Autodesk Fusion 360 part; units mm, degrees
(part 3 of 4)
  line L2118 (-48.5, -68.866) -> (-48, -69.7321)
  line L2119 (-32, -63.7321) -> (-31.5, -62.866)
  line L2120 (-47, -75.7321) -> (-46.5, -74.866)
  line L2121 (-33, -75.7321) -> (-32, -75.7321)
  line L2122 (-46.5, -74.866) -> (-47, -74)
  line L2123 (-28.5, -65.866) -> (-29, -65)
  line L2124 (-45.5, -74.866) -> (-45, -75.7321)
  line L2125 (-33, -68) -> (-33.5, -68.866)
  line L2126 (-30, -66.7321) -> (-29, -66.7321)
  line L2127 (-45.5, -71.866) -> (-45, -72.7321)
  line L2128 (-29, -68) -> (-30, -68)
  line L2129 (-47, -72.7321) -> (-46.5, -71.866)
  line L2130 (-32, -65) -> (-33, -65)
  line L2131 (-45.5, -62.866) -> (-45, -63.7321)
  line L2132 (-29, -66.7321) -> (-28.5, -65.866)
  line L2133 (-48, -75.7321) -> (-47, -75.7321)
  line L2134 (-32, -66.7321) -> (-31.5, -65.866)
  line L2135 (-48.5, -59.866) -> (-48, -60.7321)
  line L2136 (-45, -68) -> (-45.5, -68.866)
  line L2137 (-48, -72.7321) -> (-47, -72.7321)
  line L2138 (-33, -63.7321) -> (-32, -63.7321)
  line L2139 (-33, -66.7321) -> (-32, -66.7321)
  line L2140 (-33, -65) -> (-33.5, -65.866)
  line L2141 (-30, -68) -> (-30.5, -68.866)
  line L2142 (-46.5, -68.866) -> (-47, -68)
  line L2143 (-47, -74) -> (-48, -74)
  line L2144 (-47, -68) -> (-48, -68)
  line L2145 (-33, -62) -> (-33.5, -62.866)
  line L2146 (-32, -68) -> (-33, -68)
  line L2147 (-48, -74) -> (-48.5, -74.866)
  line L2148 (-48.5, -71.866) -> (-48, -72.7321)
  line L2149 (-30.5, -62.866) -> (-30, -63.7321)
  line L2150 (-48, -71) -> (-48.5, -71.866)
  line L2151 (-28.5, -62.866) -> (-29, -62)
  line L2152 (-29, -65) -> (-30, -65)
  line L2153 (-47, -69.7321) -> (-46.5, -68.866)
  line L2154 (-29, -62) -> (-30, -62)
  line L2155 (-33.5, -65.866) -> (-33, -66.7321)
  line L2156 (-30, -65) -> (-30.5, -65.866)
  line L2157 (-31.5, -68.866) -> (-32, -68)
  line L2158 (-31.5, -65.866) -> (-32, -65)
  line L2159 (-48, -65) -> (-48.5, -65.866)
  line L2160 (-28.5, -68.866) -> (-29, -68)
  line L2161 (-47, -60.7321) -> (-46.5, -59.866)
  line L2162 (-45, -59) -> (-45.5, -59.866)
  line L2163 (-33, -60.7321) -> (-32, -60.7321)
  line L2164 (-30, -60.7321) -> (-29, -60.7321)
  line L2165 (-47, -59) -> (-48, -59)
  line L2166 (-46.5, -59.866) -> (-47, -59)
  line L2167 (-46.5, -62.866) -> (-47, -62)
  line L2168 (-48, -63.7321) -> (-47, -63.7321)
  line L2169 (-48, -66.7321) -> (-47, -66.7321)
  line L2170 (-45.5, -59.866) -> (-45, -60.7321)
  line L2171 (-32, -59) -> (-33, -59)
  line L2172 (-48.5, -65.866) -> (-48, -66.7321)
  line L2173 (-47, -66.7321) -> (-46.5, -65.866)
  line L2174 (-28.5, -59.866) -> (-29, -59)
  line L2175 (-46.5, -65.866) -> (-47, -65)
  line L2176 (-30.5, -59.866) -> (-30, -60.7321)
  line L2177 (-45, -65) -> (-45.5, -65.866)
  line L2178 (-33, -59) -> (-33.5, -59.866)
  line L2179 (-47, -62) -> (-48, -62)
  line L2180 (-29, -60.7321) -> (-28.5, -59.866)
  line L2181 (-48, -62) -> (-48.5, -62.866)
  line L2182 (-30, -59) -> (-30.5, -59.866)
  line L2183 (-45, -62) -> (-45.5, -62.866)
  line L2184 (-48, -60.7321) -> (-47, -60.7321)
  line L2185 (-31.5, -59.866) -> (-32, -59)
  line L2186 (-29, -59) -> (-30, -59)
  line L2187 (-32, -60.7321) -> (-31.5, -59.866)
  line L2188 (-33.5, -59.866) -> (-33, -60.7321)
  line L2189 (-48.5, -62.866) -> (-48, -63.7321)
  line L2190 (-45.5, -65.866) -> (-45, -66.7321)
  line L2191 (-48, -59) -> (-48.5, -59.866)
  line L2192 (-47, -63.7321) -> (-46.5, -62.866)
  line L2193 (-47, -65) -> (-48, -65)
  line L2194 (-42, -72.7321) -> (-41, -72.7321)
  line L2195 (-41, -74) -> (-42, -74)
  line L2196 (-24.5, -71.866) -> (-24, -72.7321)
  line L2197 (-41, -75.7321) -> (-40.5, -74.866)
  line L2198 (-41, -72.7321) -> (-40.5, -71.866)
  line L2199 (-40.5, -68.866) -> (-41, -68)
  line L2200 (-27, -69.7321) -> (-26, -69.7321)
  line L2201 (-41, -71) -> (-42, -71)
  line L2202 (-26, -69.7321) -> (-25.5, -68.866)
  line L2203 (-43.5, -74.866) -> (-44, -74)
  line L2204 (-39.5, -71.866) -> (-39, -72.7321)
  line L2205 (-54.5, -62.866) -> (-54, -63.7321)
  line L2206 (-54, -62) -> (-54.5, -62.866)
  line L2207 (-56, -59) -> (-57, -59)
  line L2208 (-35, -72.7321) -> (-34.5, -71.866)
  line L2209 (-38, -62) -> (-39, -62)
  line L2210 (-56, -62) -> (-57, -62)
  line L2211 (-38, -72.7321) -> (-37.5, -71.866)
  line L2212 (-56, -63.7321) -> (-55.5, -62.866)
  line L2213 (-57, -60.7321) -> (-56, -60.7321)
  line L2214 (-36, -75.7321) -> (-35, -75.7321)
  line L2215 (-34.5, -71.866) -> (-35, -71)
  line L2216 (-56, -66.7321) -> (-55.5, -65.866)
  line L2217 (-36, -66.7321) -> (-35, -66.7321)
  line L2218 (-57, -59) -> (-57.5, -59.866)
  line L2219 (-39.5, -68.866) -> (-39, -69.7321)
  line L2220 (-57, -62) -> (-57.5, -62.866)
  line L2221 (-57, -66.7321) -> (-56, -66.7321)
  line L2222 (-39, -66.7321) -> (-38, -66.7321)
  line L2223 (-36, -74) -> (-36.5, -74.866)
  line L2224 (-57.5, -65.866) -> (-57, -66.7321)
  line L2225 (-36, -63.7321) -> (-35, -63.7321)
  line L2226 (-35, -63.7321) -> (-34.5, -62.866)
  line L2227 (-36, -68) -> (-36.5, -68.866)
  line L2228 (-39.5, -65.866) -> (-39, -66.7321)
  line L2229 (-57.5, -62.866) -> (-57, -63.7321)
  line L2230 (-54.5, -59.866) -> (-54, -60.7321)
  line L2231 (-38, -63.7321) -> (-37.5, -62.866)
  line L2232 (-56, -60.7321) -> (-55.5, -59.866)
  line L2233 (-54, -59) -> (-54.5, -59.866)
  line L2234 (-54.5, -65.866) -> (-54, -66.7321)
  line L2235 (-36, -62) -> (-36.5, -62.866)
  line L2236 (-36.5, -71.866) -> (-36, -72.7321)
  line L2237 (-55.5, -65.866) -> (-56, -65)
  line L2238 (-34.5, -74.866) -> (-35, -74)
  line L2239 (-57, -63.7321) -> (-56, -63.7321)
  line L2240 (-35, -71) -> (-36, -71)
  line L2241 (-36.5, -74.866) -> (-36, -75.7321)
  line L2242 (-38, -69.7321) -> (-37.5, -68.866)
  line L2243 (-39, -69.7321) -> (-38, -69.7321)
  line L2244 (-35, -75.7321) -> (-34.5, -74.866)
  line L2245 (-55.5, -59.866) -> (-56, -59)
  line L2246 (-36.5, -68.866) -> (-36, -69.7321)
  line L2247 (-54, -65) -> (-54.5, -65.866)
  line L2248 (-38, -71) -> (-39, -71)
  line L2249 (-56, -65) -> (-57, -65)
  line L2250 (-39.5, -74.866) -> (-39, -75.7321)
  line L2251 (-39, -72.7321) -> (-38, -72.7321)
  line L2252 (-39, -74) -> (-39.5, -74.866)
  line L2253 (-39, -71) -> (-39.5, -71.866)
  line L2254 (-57.5, -59.866) -> (-57, -60.7321)
  line L2255 (-35, -74) -> (-36, -74)
  line L2256 (-35, -69.7321) -> (-34.5, -68.866)
  line L2257 (-57, -65) -> (-57.5, -65.866)
  line L2258 (-36, -72.7321) -> (-35, -72.7321)
  line L2259 (-55.5, -62.866) -> (-56, -62)
  line L2260 (-59, -72.7321) -> (-58.5, -71.866)
  line L2261 (-60, -75.7321) -> (-59, -75.7321)
  line L2262 (-59, -69.7321) -> (-58.5, -68.866)
  line L2263 (-59, -74) -> (-60, -74)
  line L2264 (-60, -74) -> (-60.5, -74.866)
  line L2265 (-63.5, -68.866) -> (-63, -69.7321)
  line L2266 (-61.5, -74.866) -> (-62, -74)
  line L2267 (-60.5, -71.866) -> (-60, -72.7321)
  line L2268 (-63.5, -74.866) -> (-63, -75.7321)
  line L2269 (-60.5, -68.866) -> (-60, -69.7321)
  line L2270 (-62, -75.7321) -> (-61.5, -74.866)
  line L2271 (-60, -69.7321) -> (-59, -69.7321)
  line L2272 (-63, -71) -> (-63.5, -71.866)
  line L2273 (-60, -72.7321) -> (-59, -72.7321)
  line L2274 (-60, -71) -> (-60.5, -71.866)
  line L2275 (-63, -72.7321) -> (-62, -72.7321)
  line L2276 (-60, -66.7321) -> (-59, -66.7321)
  line L2277 (-63, -65) -> (-63.5, -65.866)
  line L2278 (-63.5, -62.866) -> (-63, -63.7321)
  line L2279 (-59, -60.7321) -> (-58.5, -59.866)
  line L2280 (-59, -66.7321) -> (-58.5, -65.866)
  line L2281 (-60, -65) -> (-60.5, -65.866)
  line L2282 (-59, -65) -> (-60, -65)
  line L2283 (-60, -59) -> (-60.5, -59.866)
  line L2284 (-62, -66.7321) -> (-61.5, -65.866)
  line L2285 (-58.5, -62.866) -> (-59, -62)
  line L2286 (-63, -68) -> (-63.5, -68.866)
  line L2287 (-60.5, -65.866) -> (-60, -66.7321)
  line L2288 (-63.5, -59.866) -> (-63, -60.7321)
  line L2289 (-60, -63.7321) -> (-59, -63.7321)
  line L2290 (-62, -68) -> (-63, -68)
  line L2291 (-61.5, -65.866) -> (-62, -65)
  line L2292 (-60, -62) -> (-60.5, -62.866)
  line L2293 (-59, -63.7321) -> (-58.5, -62.866)
  line L2294 (-58.5, -68.866) -> (-59, -68)
  line L2295 (-63, -66.7321) -> (-62, -66.7321)
  line L2296 (-62, -62) -> (-63, -62)
  line L2297 (-59, -68) -> (-60, -68)
  line L2298 (-40.5, -74.866) -> (-41, -74)
  line L2299 (-25.5, -74.866) -> (-26, -74)
  line L2300 (-27, -74) -> (-27.5, -74.866)
  line L2301 (-42.5, -74.866) -> (-42, -75.7321)
  line L2302 (-44, -75.7321) -> (-43.5, -74.866)
  line L2303 (-42.5, -68.866) -> (-42, -69.7321)
  line L2304 (-26, -68) -> (-27, -68)
  line L2305 (-43.5, -68.866) -> (-44, -68)
  line L2306 (-42, -68) -> (-42.5, -68.866)
  line L2307 (-24.5, -68.866) -> (-24, -69.7321)
  line L2308 (-44, -69.7321) -> (-43.5, -68.866)
  line L2309 (-42, -75.7321) -> (-41, -75.7321)
  line L2310 (-40.5, -71.866) -> (-41, -71)
  line L2311 (-41, -68) -> (-42, -68)
  line L2312 (-25.5, -71.866) -> (-26, -71)
  line L2313 (-27.5, -71.866) -> (-27, -72.7321)
  line L2314 (-27.5, -68.866) -> (-27, -69.7321)
  line L2315 (-27, -72.7321) -> (-26, -72.7321)
  line L2316 (-26, -74) -> (-27, -74)
  line L2317 (-43.5, -71.866) -> (-44, -71)
  line L2318 (-42, -71) -> (-42.5, -71.866)
  line L2319 (-26, -75.7321) -> (-25.5, -74.866)
  line L2320 (-27, -75.7321) -> (-26, -75.7321)
  line L2321 (-26, -71) -> (-27, -71)
  line L2322 (-42.5, -71.866) -> (-42, -72.7321)
  line L2323 (-42, -74) -> (-42.5, -74.866)
  line L2324 (-24.5, -74.866) -> (-24, -75.7321)
  line L2325 (-42, -69.7321) -> (-41, -69.7321)
  line L2326 (-27, -71) -> (-27.5, -71.866)
  line L2327 (-24, -74) -> (-24.5, -74.866)
  line L2328 (-24, -71) -> (-24.5, -71.866)
  line L2329 (-27.5, -74.866) -> (-27, -75.7321)
  line L2330 (-41, -69.7321) -> (-40.5, -68.866)
  line L2331 (-26, -72.7321) -> (-25.5, -71.866)
  line L2332 (-44, -72.7321) -> (-43.5, -71.866)
  line L2333 (-26, -66.7321) -> (-25.5, -65.866)
  line L2334 (-27, -65) -> (-27.5, -65.866)
  line L2335 (-25.5, -68.866) -> (-26, -68)
  line L2336 (-41, -65) -> (-42, -65)
  line L2337 (-44, -66.7321) -> (-43.5, -65.866)
  line L2338 (-42, -65) -> (-42.5, -65.866)
  line L2339 (-27.5, -65.866) -> (-27, -66.7321)
  line L2340 (-26, -65) -> (-27, -65)
  line L2341 (-42.5, -62.866) -> (-42, -63.7321)
  line L2342 (-26, -62) -> (-27, -62)
  line L2343 (-42, -63.7321) -> (-41, -63.7321)
  line L2344 (-41, -62) -> (-42, -62)
  line L2345 (-25.5, -65.866) -> (-26, -65)
  line L2346 (-27.5, -62.866) -> (-27, -63.7321)
  line L2347 (-42, -59) -> (-42.5, -59.866)
  line L2348 (-24, -62) -> (-24.5, -62.866)
  line L2349 (-24.5, -62.866) -> (-24, -63.7321)
  line L2350 (-43.5, -59.866) -> (-44, -59)
  line L2351 (-27, -68) -> (-27.5, -68.866)
  line L2352 (-43.5, -65.866) -> (-44, -65)
  line L2353 (-27, -66.7321) -> (-26, -66.7321)
  line L2354 (-44, -60.7321) -> (-43.5, -59.866)
  line L2355 (-42.5, -65.866) -> (-42, -66.7321)
  line L2356 (-40.5, -62.866) -> (-41, -62)
  line L2357 (-24.5, -65.866) -> (-24, -66.7321)
  line L2358 (-24, -65) -> (-24.5, -65.866)
  line L2359 (-27, -63.7321) -> (-26, -63.7321)
  line L2360 (-42, -62) -> (-42.5, -62.866)
  line L2361 (-44, -63.7321) -> (-43.5, -62.866)
  line L2362 (-24, -68) -> (-24.5, -68.866)
  line L2363 (-42.5, -59.866) -> (-42, -60.7321)
  line L2364 (-41, -63.7321) -> (-40.5, -62.866)
  line L2365 (-41, -59) -> (-42, -59)
  line L2366 (-27, -62) -> (-27.5, -62.866)
  line L2367 (-42, -60.7321) -> (-41, -60.7321)
  line L2368 (-45, -66.7321) -> (-44, -66.7321)
  line L2369 (-26, -63.7321) -> (-25.5, -62.866)
  line L2370 (-44, -65) -> (-45, -65)
  line L2371 (-45, -75.7321) -> (-44, -75.7321)
  line L2372 (-25.5, -59.866) -> (-26, -59)
  line L2373 (-24.5, -59.866) -> (-24, -60.7321)
  line L2374 (-41, -66.7321) -> (-40.5, -65.866)
  line L2375 (-45, -69.7321) -> (-44, -69.7321)
  line L2376 (-24, -59) -> (-24.5, -59.866)
  line L2377 (-44, -68) -> (-45, -68)
  line L2378 (-26, -60.7321) -> (-25.5, -59.866)
  line L2379 (-27.5, -59.866) -> (-27, -60.7321)
  line L2380 (-42, -66.7321) -> (-41, -66.7321)
  line L2381 (-44, -74) -> (-45, -74)
  line L2382 (-20, -72.7321) -> (-19.5, -71.866)
  line L2383 (-45, -60.7321) -> (-44, -60.7321)
  line L2384 (-45, -72.7321) -> (-44, -72.7321)
  line L2385 (-26, -59) -> (-27, -59)
  line L2386 (-20, -74) -> (-21, -74)
  line L2387 (-25.5, -62.866) -> (-26, -62)
  line L2388 (-40.5, -65.866) -> (-41, -65)
  line L2389 (-40.5, -59.866) -> (-41, -59)
  line L2390 (-43.5, -62.866) -> (-44, -62)
  line L2391 (-41, -60.7321) -> (-40.5, -59.866)
  line L2392 (-44, -62) -> (-45, -62)
  line L2393 (-27, -60.7321) -> (-26, -60.7321)
  line L2394 (-45, -63.7321) -> (-44, -63.7321)
  line L2395 (-44, -59) -> (-45, -59)
  line L2396 (-27, -59) -> (-27.5, -59.866)
  line L2397 (-44, -71) -> (-45, -71)
  line L2398 (-21, -71) -> (-21.5, -71.866)
  line L2399 (-21, -72.7321) -> (-20, -72.7321)
  line L2400 (-20, -69.7321) -> (-19.5, -68.866)
  line L2401 (-21, -75.7321) -> (-20, -75.7321)
  line L2402 (-23, -75.7321) -> (-22.5, -74.866)
  line L2403 (-21.5, -71.866) -> (-21, -72.7321)
  line L2404 (-21.5, -68.866) -> (-21, -69.7321)
  line L2405 (-21.5, -74.866) -> (-21, -75.7321)
  line L2406 (-21, -69.7321) -> (-20, -69.7321)
  line L2407 (-24, -66.7321) -> (-23, -66.7321)
  line L2408 (-16.5, -65.866) -> (-17, -65)
  line L2409 (-17, -60.7321) -> (-16.5, -59.866)
  line L2410 (-18, -62) -> (-18.5, -62.866)
  line L2411 (-24, -75.7321) -> (-23, -75.7321)
  line L2412 (-15, -62) -> (-15.5, -62.866)
  line L2413 (-18, -65) -> (-18.5, -65.866)
  line L2414 (-15, -65) -> (-15.5, -65.866)
  line L2415 (-23, -65) -> (-24, -65)
  line L2416 (-17, -63.7321) -> (-16.5, -62.866)
  line L2417 (-18, -60.7321) -> (-17, -60.7321)
  line L2418 (-18, -68) -> (-18.5, -68.866)
  line L2419 (-15.5, -59.866) -> (-15, -60.7321)
  line L2420 (-24, -69.7321) -> (-23, -69.7321)
  line L2421 (-18, -63.7321) -> (-17, -63.7321)
  line L2422 (-16.5, -68.866) -> (-17, -68)
  line L2423 (-15.5, -65.866) -> (-15, -66.7321)
  line L2424 (-17, -68) -> (-18, -68)
  line L2425 (-18, -59) -> (-18.5, -59.866)
  line L2426 (-22.5, -74.866) -> (-23, -74)
  line L2427 (-21.5, -62.866) -> (-21, -63.7321)
  line L2428 (-20, -71) -> (-21, -71)
  line L2429 (-22.5, -71.866) -> (-23, -71)
  line L2430 (-19.5, -74.866) -> (-20, -74)
  line L2431 (-21, -68) -> (-21.5, -68.866)
  line L2432 (-19.5, -71.866) -> (-20, -71)
  line L2433 (-22.5, -62.866) -> (-23, -62)
  line L2434 (-15, -74) -> (-15.5, -74.866)
  line L2435 (-19.5, -68.866) -> (-20, -68)
  line L2436 (-20, -68) -> (-21, -68)
  line L2437 (-23, -72.7321) -> (-22.5, -71.866)
  line L2438 (-20, -75.7321) -> (-19.5, -74.866)
  line L2439 (-21, -62) -> (-21.5, -62.866)
  line L2440 (-23, -69.7321) -> (-22.5, -68.866)
  line L2441 (-21, -74) -> (-21.5, -74.866)
  line L2442 (-17, -75.7321) -> (-16.5, -74.866)
  line L2443 (-20, -66.7321) -> (-19.5, -65.866)
  line L2444 (-18, -69.7321) -> (-17, -69.7321)
  line L2445 (-19.5, -62.866) -> (-20, -62)
  line L2446 (-18.5, -71.866) -> (-18, -72.7321)
  line L2447 (-18, -74) -> (-18.5, -74.866)
  line L2448 (-15, -71) -> (-15.5, -71.866)
  line L2449 (-21, -59) -> (-21.5, -59.866)
  line L2450 (-17, -72.7321) -> (-16.5, -71.866)
  line L2451 (-20, -59) -> (-21, -59)
  line L2452 (-22.5, -65.866) -> (-23, -65)
  line L2453 (-21.5, -65.866) -> (-21, -66.7321)
  line L2454 (-21, -63.7321) -> (-20, -63.7321)
  line L2455 (-17, -74) -> (-18, -74)
  line L2456 (-21, -66.7321) -> (-20, -66.7321)
  line L2457 (-23, -63.7321) -> (-22.5, -62.866)
  line L2458 (-20, -62) -> (-21, -62)
  line L2459 (-15.5, -74.866) -> (-15, -75.7321)
  line L2460 (-18, -71) -> (-18.5, -71.866)
  line L2461 (-16.5, -71.866) -> (-17, -71)
  line L2462 (-19.5, -65.866) -> (-20, -65)
  line L2463 (-19.5, -59.866) -> (-20, -59)
  line L2464 (-18.5, -68.866) -> (-18, -69.7321)
  line L2465 (-23, -60.7321) -> (-22.5, -59.866)
  line L2466 (-18.5, -62.866) -> (-18, -63.7321)
  line L2467 (-20, -65) -> (-21, -65)
  line L2468 (-16.5, -74.866) -> (-17, -74)
  line L2469 (-18, -75.7321) -> (-17, -75.7321)
  line L2470 (-17, -71) -> (-18, -71)
  line L2471 (-15.5, -68.866) -> (-15, -69.7321)
  line L2472 (-21, -65) -> (-21.5, -65.866)
  line L2473 (-20, -63.7321) -> (-19.5, -62.866)
  line L2474 (-15.5, -71.866) -> (-15, -72.7321)
  line L2475 (-18, -72.7321) -> (-17, -72.7321)
  line L2476 (-22.5, -68.866) -> (-23, -68)
  line L2477 (-18.5, -74.866) -> (-18, -75.7321)
  line L2478 (-17, -69.7321) -> (-16.5, -68.866)
  line L2479 (-23, -66.7321) -> (-22.5, -65.866)
  line L2480 (-22.5, -59.866) -> (-23, -59)
  line L2481 (-20, -60.7321) -> (-19.5, -59.866)
  line L2482 (-17, -65) -> (-18, -65)
  line L2483 (-17, -62) -> (-18, -62)
  line L2484 (-15.5, -62.866) -> (-15, -63.7321)
  line L2485 (-24, -63.7321) -> (-23, -63.7321)
  line L2486 (-16.5, -62.866) -> (-17, -62)
  line L2487 (-23, -59) -> (-24, -59)
  line L2488 (-15, -68) -> (-15.5, -68.866)
  line L2489 (-23, -62) -> (-24, -62)
  line L2490 (-23, -71) -> (-24, -71)
  line L2491 (-21, -60.7321) -> (-20, -60.7321)
  line L2492 (-24, -60.7321) -> (-23, -60.7321)
  line L2493 (-24, -72.7321) -> (-23, -72.7321)
  line L2494 (-23, -68) -> (-24, -68)
  line L2495 (-18.5, -65.866) -> (-18, -66.7321)
  line L2496 (-21.5, -59.866) -> (-21, -60.7321)
  line L2497 (-23, -74) -> (-24, -74)
  line L2498 (-18, -66.7321) -> (-17, -66.7321)
  line L2499 (-17, -66.7321) -> (-16.5, -65.866)
  line L2500 (-49.5, -65.866) -> (-50, -65)
  line L2501 (-37.5, -68.866) -> (-38, -68)
  line L2502 (-39, -60.7321) -> (-38, -60.7321)
  line L2503 (-51.5, -65.866) -> (-51, -66.7321)
  line L2504 (-34.5, -59.866) -> (-35, -59)
  line L2505 (-38, -59) -> (-39, -59)
  line L2506 (-50, -59) -> (-51, -59)
  line L2507 (-36.5, -65.866) -> (-36, -66.7321)
  line L2508 (-51, -74) -> (-51.5, -74.866)
  line L2509 (-52.5, -68.866) -> (-53, -68)
  line L2510 (-49.5, -68.866) -> (-50, -68)
  line L2511 (-53, -72.7321) -> (-52.5, -71.866)
  line L2512 (-35, -66.7321) -> (-34.5, -65.866)
  line L2513 (-35, -65) -> (-36, -65)
  line L2514 (-50, -75.7321) -> (-49.5, -74.866)
  line L2515 (-51, -69.7321) -> (-50, -69.7321)
  line L2516 (-52.5, -71.866) -> (-53, -71)
  line L2517 (-35, -60.7321) -> (-34.5, -59.866)
  line L2518 (-39, -65) -> (-39.5, -65.866)
  line L2519 (-36, -59) -> (-36.5, -59.866)
  line L2520 (-35, -59) -> (-36, -59)
  line L2521 (-37.5, -62.866) -> (-38, -62)
  line L2522 (-39, -68) -> (-39.5, -68.866)
  line L2523 (-51.5, -68.866) -> (-51, -69.7321)
  line L2524 (-53, -60.7321) -> (-52.5, -59.866)
  line L2525 (-51.5, -74.866) -> (-51, -75.7321)
  line L2526 (-39, -59) -> (-39.5, -59.866)
  line L2527 (-36.5, -59.866) -> (-36, -60.7321)
  line L2528 (-50, -62) -> (-51, -62)
  line L2529 (-38, -60.7321) -> (-37.5, -59.866)
  line L2530 (-49.5, -74.866) -> (-50, -74)
  line L2531 (-49.5, -71.866) -> (-50, -71)
  line L2532 (-35, -62) -> (-36, -62)
  line L2533 (-38, -68) -> (-39, -68)
  line L2534 (-36, -65) -> (-36.5, -65.866)
  line L2535 (-36.5, -62.866) -> (-36, -63.7321)
  line L2536 (-53, -69.7321) -> (-52.5, -68.866)
  line L2537 (-34.5, -68.866) -> (-35, -68)
  line L2538 (-50, -72.7321) -> (-49.5, -71.866)
  line L2539 (-51, -68) -> (-51.5, -68.866)
  line L2540 (-35, -68) -> (-36, -68)
  line L2541 (-51, -71) -> (-51.5, -71.866)
  line L2542 (-37.5, -65.866) -> (-38, -65)
  line L2543 (-50, -68) -> (-51, -68)
  line L2544 (-39, -63.7321) -> (-38, -63.7321)
  line L2545 (-50, -74) -> (-51, -74)
  line L2546 (-38, -66.7321) -> (-37.5, -65.866)
  line L2547 (-34.5, -65.866) -> (-35, -65)
  line L2548 (-39.5, -62.866) -> (-39, -63.7321)
  line L2549 (-51, -75.7321) -> (-50, -75.7321)
  line L2550 (-50, -69.7321) -> (-49.5, -68.866)
  line L2551 (-51.5, -71.866) -> (-51, -72.7321)
  line L2552 (-52.5, -74.866) -> (-53, -74)
  line L2553 (-39, -62) -> (-39.5, -62.866)
  line L2554 (-38, -65) -> (-39, -65)
  line L2555 (-50, -71) -> (-51, -71)
  line L2556 (-34.5, -62.866) -> (-35, -62)
  line L2557 (-51, -72.7321) -> (-50, -72.7321)
  line L2558 (-53, -75.7321) -> (-52.5, -74.866)
  line L2559 (-51, -60.7321) -> (-50, -60.7321)
  line L2560 (-32, -71) -> (-33, -71)
  line L2561 (-32, -72.7321) -> (-31.5, -71.866)
  line L2562 (-30.5, -71.866) -> (-30, -72.7321)
  line L2563 (-51.5, -59.866) -> (-51, -60.7321)
  line L2564 (-49.5, -62.866) -> (-50, -62)
  line L2565 (-36, -60.7321) -> (-35, -60.7321)
  line L2566 (-52.5, -65.866) -> (-53, -65)
  line L2567 (-37.5, -59.866) -> (-38, -59)
  line L2568 (-51.5, -62.866) -> (-51, -63.7321)
  line L2569 (-52.5, -59.866) -> (-53, -59)
  line L2570 (-51, -59) -> (-51.5, -59.866)
  line L2571 (-33, -71) -> (-33.5, -71.866)
  line L2572 (-30.5, -74.866) -> (-30, -75.7321)
  line L2573 (-51, -66.7321) -> (-50, -66.7321)
  line L2574 (-52.5, -62.866) -> (-53, -62)
  line L2575 (-51, -62) -> (-51.5, -62.866)
  line L2576 (-29, -75.7321) -> (-28.5, -74.866)
  line L2577 (-53, -71) -> (-54, -71)
  line L2578 (-53, -66.7321) -> (-52.5, -65.866)
  line L2579 (-30, -69.7321) -> (-29, -69.7321)
  line L2580 (-51, -63.7321) -> (-50, -63.7321)
  line L2581 (-51, -65) -> (-51.5, -65.866)
  line L2582 (-50, -65) -> (-51, -65)
  line L2583 (-50, -66.7321) -> (-49.5, -65.866)
  line L2584 (-39.5, -59.866) -> (-39, -60.7321)
  line L2585 (-49.5, -59.866) -> (-50, -59)
  line L2586 (-29, -71) -> (-30, -71)
  line L2587 (-50, -63.7321) -> (-49.5, -62.866)
  line L2588 (-32, -74) -> (-33, -74)
  line L2589 (-50, -60.7321) -> (-49.5, -59.866)
  line L2590 (-53, -63.7321) -> (-52.5, -62.866)
  line L2591 (-30, -72.7321) -> (-29, -72.7321)
  line L2592 (-33.5, -71.866) -> (-33, -72.7321)
  line L2593 (-53, -59) -> (-54, -59)
  line L2594 (-54, -63.7321) -> (-53, -63.7321)
  line L2595 (-53, -65) -> (-54, -65)
  line L2596 (-31.5, -74.866) -> (-32, -74)
  line L2597 (-53, -74) -> (-54, -74)
  line L2598 (-54, -72.7321) -> (-53, -72.7321)
  line L2599 (-53, -62) -> (-54, -62)
  line L2600 (-28.5, -74.866) -> (-29, -74)
  line L2601 (-30.5, -68.866) -> (-30, -69.7321)
  line L2602 (-28.5, -71.866) -> (-29, -71)
  line L2603 (-33, -72.7321) -> (-32, -72.7321)
  line L2604 (-29, -69.7321) -> (-28.5, -68.866)
  line L2605 (-32, -75.7321) -> (-31.5, -74.866)
  line L2606 (-54, -66.7321) -> (-53, -66.7321)
  line L2607 (-30, -74) -> (-30.5, -74.866)
  line L2608 (-32, -69.7321) -> (-31.5, -68.866)
  line L2609 (-30, -71) -> (-30.5, -71.866)
  line L2610 (-54, -69.7321) -> (-53, -69.7321)
  line L2611 (-54, -60.7321) -> (-53, -60.7321)
  line L2612 (-30, -75.7321) -> (-29, -75.7321)
  line L2613 (-33, -74) -> (-33.5, -74.866)
  line L2614 (-54, -75.7321) -> (-53, -75.7321)
  line L2615 (-33.5, -74.866) -> (-33, -75.7321)
  line L2616 (-31.5, -71.866) -> (-32, -71)
  line L2617 (-53, -68) -> (-54, -68)
  line L2618 (-29, -74) -> (-30, -74)
  line L2619 (-17, -59) -> (-18, -59)
  line L2620 (-15, -59) -> (-15.5, -59.866)
  line L2621 (-18.5, -59.866) -> (-18, -60.7321)
  line L2622 (-16.5, -59.866) -> (-17, -59)
  line L2623 (-63.5, -65.866) -> (-63, -66.7321)
  line L2624 (-63, -63.7321) -> (-62, -63.7321)
  line L2625 (-59, -62) -> (-60, -62)
  line L2626 (-63, -62) -> (-63.5, -62.866)
  line L2627 (-61.5, -68.866) -> (-62, -68)
  line L2628 (-62, -65) -> (-63, -65)
  line L2629 (-62, -63.7321) -> (-61.5, -62.866)
  line L2630 (-60, -68) -> (-60.5, -68.866)
  line L2631 (-61.5, -62.866) -> (-62, -62)
  line L2632 (-58.5, -65.866) -> (-59, -65)
  line L2633 (-60.5, -62.866) -> (-60, -63.7321)
  line L2634 (-61.5, -71.866) -> (-62, -71)
  line L2635 (-58.5, -74.866) -> (-59, -74)
  line L2636 (-63, -69.7321) -> (-62, -69.7321)
  line L2637 (-58.5, -71.866) -> (-59, -71)
  line L2638 (-63, -75.7321) -> (-62, -75.7321)
  line L2639 (-63, -74) -> (-63.5, -74.866)
  line L2640 (-63.5, -71.866) -> (-63, -72.7321)
  line L2641 (-59, -71) -> (-60, -71)
  line L2642 (-62, -71) -> (-63, -71)
  line L2643 (-62, -69.7321) -> (-61.5, -68.866)
  line L2644 (-12.5, -80.866) -> (-12, -81.7321)
  line L2645 (-10.5, -80.866) -> (-11, -80)
  line L2646 (-12, -77) -> (-12.5, -77.866)
  line L2647 (-17, -78.7321) -> (-16.5, -77.866)
  line L2648 (-44, -80) -> (-45, -80)
  line L2649 (-18, -78.7321) -> (-17, -78.7321)
  line L2650 (-22.5, -80.866) -> (-23, -80)
  line L2651 (-41, -77) -> (-42, -77)
  line L2652 (-21, -80) -> (-21.5, -80.866)
  line L2653 (-20, -81.7321) -> (-19.5, -80.866)
  line L2654 (-44, -78.7321) -> (-43.5, -77.866)
  line L2655 (-16.5, -80.866) -> (-17, -80)
  line L2656 (-21, -77) -> (-21.5, -77.866)
  line L2657 (-41, -81.7321) -> (-40.5, -80.866)
  line L2658 (-12.5, -77.866) -> (-12, -78.7321)
  line L2659 (-23, -77) -> (-24, -77)
  line L2660 (-20, -77) -> (-21, -77)
  line L2661 (-22.5, -77.866) -> (-23, -77)
  line L2662 (-24, -78.7321) -> (-23, -78.7321)
  line L2663 (-23, -78.7321) -> (-22.5, -77.866)
  line L2664 (-23, -80) -> (-24, -80)
  line L2665 (-44, -81.7321) -> (-43.5, -80.866)
  line L2666 (-20, -78.7321) -> (-19.5, -77.866)
  line L2667 (-20, -80) -> (-21, -80)
  line L2668 (-42, -77) -> (-42.5, -77.866)
  line L2669 (-42, -81.7321) -> (-41, -81.7321)
  line L2670 (-15.5, -77.866) -> (-15, -78.7321)
  line L2671 (-18, -80) -> (-18.5, -80.866)
  line L2672 (-42, -80) -> (-42.5, -80.866)
  line L2673 (-21, -78.7321) -> (-20, -78.7321)
  line L2674 (-17, -80) -> (-18, -80)
  line L2675 (-21.5, -77.866) -> (-21, -78.7321)
  line L2676 (-40.5, -77.866) -> (-41, -77)
  line L2677 (-15.5, -80.866) -> (-15, -81.7321)
  line L2678 (-19.5, -80.866) -> (-20, -80)
  line L2679 (-18.5, -80.866) -> (-18, -81.7321)
  line L2680 (-15, -77) -> (-15.5, -77.866)
  line L2681 (-40.5, -80.866) -> (-41, -80)
  line L2682 (-17, -77) -> (-18, -77)
  line L2683 (-12, -80) -> (-12.5, -80.866)
  line L2684 (-11, -81.7321) -> (-10.5, -80.866)
  line L2685 (-11, -80) -> (-12, -80)
  line L2686 (-21.5, -80.866) -> (-21, -81.7321)
  line L2687 (-18, -81.7321) -> (-17, -81.7321)
  line L2688 (-24, -81.7321) -> (-23, -81.7321)
  line L2689 (-45, -78.7321) -> (-44, -78.7321)
  line L2690 (-21, -81.7321) -> (-20, -81.7321)
  line L2691 (-23, -81.7321) -> (-22.5, -80.866)
  line L2692 (-18, -77) -> (-18.5, -77.866)
  line L2693 (-44, -77) -> (-45, -77)
  line L2694 (-19.5, -77.866) -> (-20, -77)
  line L2695 (-10.5, -77.866) -> (-11, -77)
  line L2696 (-14, -78.7321) -> (-13.5, -77.866)
  line L2697 (-13.5, -77.866) -> (-14, -77)
  line L2698 (-11, -77) -> (-12, -77)
  line L2699 (-11, -78.7321) -> (-10.5, -77.866)
  line L2700 (-12, -78.7321) -> (-11, -78.7321)
  line L2701 (-13.5, -80.866) -> (-14, -80)
  line L2702 (-12, -81.7321) -> (-11, -81.7321)
  line L2703 (-14, -77) -> (-15, -77)
  line L2704 (-15, -81.7321) -> (-14, -81.7321)
  line L2705 (-14, -81.7321) -> (-13.5, -80.866)
  line L2706 (-15, -78.7321) -> (-14, -78.7321)
  line L2707 (-14, -80) -> (-15, -80)
  line L2708 (-35, -81.7321) -> (-34.5, -80.866)
  line L2709 (-57, -80) -> (-57.5, -80.866)
  line L2710 (-35, -77) -> (-36, -77)
  line L2711 (-57, -77) -> (-57.5, -77.866)
  line L2712 (-54, -77) -> (-54.5, -77.866)
  line L2713 (-63, -78.7321) -> (-62, -78.7321)
  line L2714 (-60.5, -77.866) -> (-60, -78.7321)
  line L2715 (-59, -81.7321) -> (-58.5, -80.866)
  line L2716 (-63, -80) -> (-63.5, -80.866)
  line L2717 (-63.5, -77.866) -> (-63, -78.7321)
  line L2718 (-63, -81.7321) -> (-62, -81.7321)
  line L2719 (-60, -77) -> (-60.5, -77.866)
  line L2720 (-59, -80) -> (-60, -80)
  line L2721 (-60.5, -80.866) -> (-60, -81.7321)
  line L2722 (-59, -77) -> (-60, -77)
  line L2723 (-62, -78.7321) -> (-61.5, -77.866)
  line L2724 (-62, -80) -> (-63, -80)
  line L2725 (-61.5, -77.866) -> (-62, -77)
  line L2726 (-58.5, -77.866) -> (-59, -77)
  line L2727 (-63.5, -80.866) -> (-63, -81.7321)
  line L2728 (-60, -78.7321) -> (-59, -78.7321)
  line L2729 (-62, -77) -> (-63, -77)
  line L2730 (-60, -81.7321) -> (-59, -81.7321)
  line L2731 (-63, -77) -> (-63.5, -77.866)
  line L2732 (-61.5, -80.866) -> (-62, -80)
  line L2733 (-62, -81.7321) -> (-61.5, -80.866)
  line L2734 (-58.5, -80.866) -> (-59, -80)
  line L2735 (-60, -80) -> (-60.5, -80.866)
  line L2736 (-59, -78.7321) -> (-58.5, -77.866)
  line L2737 (-68, -77) -> (-69, -77)
  line L2738 (-69, -77) -> (-69.5, -77.866)
  line L2739 (-65, -78.7321) -> (-64.5, -77.866)
  line L2740 (-66, -81.7321) -> (-65, -81.7321)
  line L2741 (-69, -81.7321) -> (-68, -81.7321)
  line L2742 (-66.5, -77.866) -> (-66, -78.7321)
  line L2743 (-68, -81.7321) -> (-67.5, -80.866)
  line L2744 (-66, -80) -> (-66.5, -80.866)
  line L2745 (-66, -77) -> (-66.5, -77.866)
  line L2746 (-65, -77) -> (-66, -77)
  line L2747 (-68, -80) -> (-69, -80)
  line L2748 (-65, -81.7321) -> (-64.5, -80.866)
  line L2749 (-66.5, -80.866) -> (-66, -81.7321)
  line L2750 (-65, -80) -> (-66, -80)
  line L2751 (-66, -78.7321) -> (-65, -78.7321)
  line L2752 (-64.5, -77.866) -> (-65, -77)
  line L2753 (-69.5, -80.866) -> (-69, -81.7321)
  line L2754 (-69.5, -77.866) -> (-69, -78.7321)
  line L2755 (-67.5, -80.866) -> (-68, -80)
  line L2756 (-69, -78.7321) -> (-68, -78.7321)
  line L2757 (-68, -78.7321) -> (-67.5, -77.866)
  line L2758 (-69, -80) -> (-69.5, -80.866)
  line L2759 (-64.5, -80.866) -> (-65, -80)
  line L2760 (-57.5, -77.866) -> (-57, -78.7321)
  line L2761 (-57, -78.7321) -> (-56, -78.7321)
  line L2762 (-56, -78.7321) -> (-55.5, -77.866)
  line L2763 (-39.5, -80.866) -> (-39, -81.7321)
  line L2764 (-55.5, -80.866) -> (-56, -80)
  line L2765 (-39, -81.7321) -> (-38, -81.7321)
  line L2766 (-38, -77) -> (-39, -77)
  line L2767 (-55.5, -77.866) -> (-56, -77)
  line L2768 (-56, -81.7321) -> (-55.5, -80.866)
  line L2769 (-56, -77) -> (-57, -77)
  line L2770 (-54.5, -80.866) -> (-54, -81.7321)
  line L2771 (-67.5, -77.866) -> (-68, -77)
  line L2772 (-36, -78.7321) -> (-35, -78.7321)
  line L2773 (-57, -81.7321) -> (-56, -81.7321)
  line L2774 (-54, -80) -> (-54.5, -80.866)
  line L2775 (-35, -80) -> (-36, -80)
  line L2776 (-57.5, -80.866) -> (-57, -81.7321)
  line L2777 (-54.5, -77.866) -> (-54, -78.7321)
  line L2778 (-39, -78.7321) -> (-38, -78.7321)
  line L2779 (-56, -80) -> (-57, -80)
  line L2780 (-51.5, -77.866) -> (-51, -78.7321)
  line L2781 (-54, -78.7321) -> (-53, -78.7321)
  line L2782 (-39.5, -77.866) -> (-39, -78.7321)
  line L2783 (-50, -81.7321) -> (-49.5, -80.866)
  line L2784 (-33, -78.7321) -> (-32, -78.7321)
  line L2785 (-53, -81.7321) -> (-52.5, -80.866)
  line L2786 (-53, -80) -> (-54, -80)
  line L2787 (-33.5, -77.866) -> (-33, -78.7321)
  line L2788 (-30.5, -77.866) -> (-30, -78.7321)
  line L2789 (-31.5, -77.866) -> (-32, -77)
  line L2790 (-30, -81.7321) -> (-29, -81.7321)
  line L2791 (-30, -80) -> (-30.5, -80.866)
  line L2792 (-28.5, -80.866) -> (-29, -80)
  line L2793 (-49.5, -80.866) -> (-50, -80)
  line L2794 (-51, -80) -> (-51.5, -80.866)
  line L2795 (-36, -80) -> (-36.5, -80.866)
  line L2796 (-50, -78.7321) -> (-49.5, -77.866)
  line L2797 (-36, -81.7321) -> (-35, -81.7321)
  line L2798 (-49.5, -77.866) -> (-50, -77)
  line L2799 (-36, -77) -> (-36.5, -77.866)
  line L2800 (-51, -81.7321) -> (-50, -81.7321)
  line L2801 (-36.5, -77.866) -> (-36, -78.7321)
  line L2802 (-51.5, -80.866) -> (-51, -81.7321)
  line L2803 (-35, -78.7321) -> (-34.5, -77.866)
  line L2804 (-51, -77) -> (-51.5, -77.866)
  line L2805 (-50, -80) -> (-51, -80)
  line L2806 (-50, -77) -> (-51, -77)
  line L2807 (-37.5, -80.866) -> (-38, -80)
  line L2808 (-51, -78.7321) -> (-50, -78.7321)
  line L2809 (-53, -78.7321) -> (-52.5, -77.866)
  line L2810 (-39, -80) -> (-39.5, -80.866)
  line L2811 (-52.5, -77.866) -> (-53, -77)
  line L2812 (-52.5, -80.866) -> (-53, -80)
  line L2813 (-53, -77) -> (-54, -77)
  line L2814 (-54, -81.7321) -> (-53, -81.7321)
  line L2815 (-33, -80) -> (-33.5, -80.866)
  line L2816 (-30, -77) -> (-30.5, -77.866)
  line L2817 (-29, -81.7321) -> (-28.5, -80.866)
  line L2818 (-33, -81.7321) -> (-32, -81.7321)
  line L2819 (-32, -80) -> (-33, -80)
  line L2820 (-47, -77) -> (-48, -77)
  line L2821 (-30, -78.7321) -> (-29, -78.7321)
  line L2822 (-30.5, -80.866) -> (-30, -81.7321)
  line L2823 (-32, -81.7321) -> (-31.5, -80.866)
  line L2824 (-46.5, -80.866) -> (-47, -80)
  line L2825 (-29, -78.7321) -> (-28.5, -77.866)
  line L2826 (-31.5, -80.866) -> (-32, -80)
  line L2827 (-45, -81.7321) -> (-44, -81.7321)
  line L2828 (-45.5, -77.866) -> (-45, -78.7321)
  line L2829 (-32, -77) -> (-33, -77)
  line L2830 (-33.5, -80.866) -> (-33, -81.7321)
  line L2831 (-45, -80) -> (-45.5, -80.866)
  line L2832 (-29, -80) -> (-30, -80)
  line L2833 (-48.5, -77.866) -> (-48, -78.7321)
  line L2834 (-28.5, -77.866) -> (-29, -77)
  line L2835 (-46.5, -77.866) -> (-47, -77)
  line L2836 (-33, -77) -> (-33.5, -77.866)
  line L2837 (-42.5, -77.866) -> (-42, -78.7321)
  line L2838 (-18.5, -77.866) -> (-18, -78.7321)
  line L2839 (-47, -81.7321) -> (-46.5, -80.866)
  line L2840 (-43.5, -80.866) -> (-44, -80)
  line L2841 (-45, -77) -> (-45.5, -77.866)
  line L2842 (-26, -81.7321) -> (-25.5, -80.866)
  line L2843 (-47, -78.7321) -> (-46.5, -77.866)
  line L2844 (-48, -78.7321) -> (-47, -78.7321)
  line L2845 (-26, -78.7321) -> (-25.5, -77.866)
  line L2846 (-48, -81.7321) -> (-47, -81.7321)
  line L2847 (-25.5, -77.866) -> (-26, -77)
  line L2848 (-25.5, -80.866) -> (-26, -80)
  line L2849 (-42.5, -80.866) -> (-42, -81.7321)
  line L2850 (-15, -80) -> (-15.5, -80.866)
  line L2851 (-43.5, -77.866) -> (-44, -77)
  line L2852 (-41, -78.7321) -> (-40.5, -77.866)
  line L2853 (-47, -80) -> (-48, -80)
  line L2854 (-24, -80) -> (-24.5, -80.866)
  line L2855 (-24.5, -77.866) -> (-24, -78.7321)
  line L2856 (-29, -77) -> (-30, -77)
  line L2857 (-24.5, -80.866) -> (-24, -81.7321)
  line L2858 (-27, -81.7321) -> (-26, -81.7321)
  line L2859 (-26, -77) -> (-27, -77)
  line L2860 (-45.5, -80.866) -> (-45, -81.7321)
  line L2861 (-32, -78.7321) -> (-31.5, -77.866)
  line L2862 (-48, -77) -> (-48.5, -77.866)
  line L2863 (-27, -77) -> (-27.5, -77.866)
  line L2864 (-27, -78.7321) -> (-26, -78.7321)
  line L2865 (-27, -80) -> (-27.5, -80.866)
  line L2866 (-26, -80) -> (-27, -80)
  line L2867 (-48.5, -80.866) -> (-48, -81.7321)
  line L2868 (-48, -80) -> (-48.5, -80.866)
  line L2869 (-27.5, -80.866) -> (-27, -81.7321)
  line L2870 (-27.5, -77.866) -> (-27, -78.7321)
  line L2871 (-24, -77) -> (-24.5, -77.866)
  line L2872 (-17, -81.7321) -> (-16.5, -80.866)
  line L2873 (-42, -78.7321) -> (-41, -78.7321)
  line L2874 (-41, -80) -> (-42, -80)
  line L2875 (-16.5, -77.866) -> (-17, -77)
  line L2876 (-36.5, -80.866) -> (-36, -81.7321)
  line L2877 (-38, -80) -> (-39, -80)
  line L2878 (-38, -81.7321) -> (-37.5, -80.866)
  line L2879 (-34.5, -77.866) -> (-35, -77)
  line L2880 (-38, -78.7321) -> (-37.5, -77.866)
  line L2881 (-34.5, -80.866) -> (-35, -80)
  line L2882 (-37.5, -77.866) -> (-38, -77)
  line L2883 (-39, -77) -> (-39.5, -77.866)
  line L2884 (-37.5, -86.866) -> (-38, -86)
  line L2885 (-35, -84.7321) -> (-34.5, -83.866)
  line L2886 (-39, -86) -> (-39.5, -86.866)
  line L2887 (-36.5, -83.866) -> (-36, -84.7321)
  line L2888 (-36, -87.7321) -> (-35, -87.7321)
  line L2889 (-38, -86) -> (-39, -86)
  line L2890 (-35, -87.7321) -> (-34.5, -86.866)
  line L2891 (-39.5, -83.866) -> (-39, -84.7321)
  line L2892 (-34.5, -86.866) -> (-35, -86)
  line L2893 (-39.5, -86.866) -> (-39, -87.7321)
  line L2894 (-36, -84.7321) -> (-35, -84.7321)
  line L2895 (-39, -84.7321) -> (-38, -84.7321)
  line L2896 (-42, -87.7321) -> (-41, -87.7321)
  line L2897 (-42.5, -83.866) -> (-42, -84.7321)
  line L2898 (-40.5, -86.866) -> (-41, -86)
  line L2899 (-42, -84.7321) -> (-41, -84.7321)
  line L2900 (-44, -84.7321) -> (-43.5, -83.866)
  line L2901 (-42, -83) -> (-42.5, -83.866)
  line L2902 (-42, -86) -> (-42.5, -86.866)
  line L2903 (-43.5, -83.866) -> (-44, -83)
  line L2904 (-41, -87.7321) -> (-40.5, -86.866)
  line L2905 (-42.5, -86.866) -> (-42, -87.7321)
  line L2906 (-41, -83) -> (-42, -83)
  line L2907 (-36.5, -86.866) -> (-36, -87.7321)
  line L2908 (-38, -84.7321) -> (-37.5, -83.866)
  line L2909 (-35, -83) -> (-36, -83)
  line L2910 (-35, -86) -> (-36, -86)
  line L2911 (-45, -87.7321) -> (-44, -87.7321)
  line L2912 (-44, -86) -> (-45, -86)
  line L2913 (-44, -83) -> (-45, -83)
  line L2914 (-45, -84.7321) -> (-44, -84.7321)
  line L2915 (-43.5, -86.866) -> (-44, -86)
  line L2916 (-41, -86) -> (-42, -86)
  line L2917 (-41, -84.7321) -> (-40.5, -83.866)
  line L2918 (-15, -86) -> (-15.5, -86.866)
  line L2919 (-33, -86) -> (-33.5, -86.866)
  line L2920 (-38, -87.7321) -> (-37.5, -86.866)
  line L2921 (-26, -83) -> (-27, -83)
  line L2922 (-34.5, -83.866) -> (-35, -83)
  line L2923 (-27, -86) -> (-27.5, -86.866)
  line L2924 (-15.5, -83.866) -> (-15, -84.7321)
  line L2925 (-27.5, -86.866) -> (-27, -87.7321)
  line L2926 (-16.5, -86.866) -> (-17, -86)
  line L2927 (-24.5, -83.866) -> (-24, -84.7321)
  line L2928 (-15.5, -86.866) -> (-15, -87.7321)
  line L2929 (-27, -84.7321) -> (-26, -84.7321)
  line L2930 (-25.5, -86.866) -> (-26, -86)
  line L2931 (-27.5, -83.866) -> (-27, -84.7321)
  line L2932 (-24, -83) -> (-24.5, -83.866)
  line L2933 (-15, -83) -> (-15.5, -83.866)
  line L2934 (-26, -86) -> (-27, -86)
  line L2935 (-27, -87.7321) -> (-26, -87.7321)
  line L2936 (-36, -83) -> (-36.5, -83.866)
  line L2937 (-38, -83) -> (-39, -83)
  line L2938 (-27, -83) -> (-27.5, -83.866)
  line L2939 (-17, -84.7321) -> (-16.5, -83.866)
  line L2940 (-25.5, -83.866) -> (-26, -83)
  line L2941 (-37.5, -83.866) -> (-38, -83)
  line L2942 (-39, -83) -> (-39.5, -83.866)
  line L2943 (-26, -84.7321) -> (-25.5, -83.866)
  line L2944 (-18.5, -83.866) -> (-18, -84.7321)
  line L2945 (-31.5, -83.866) -> (-32, -83)
  line L2946 (-39, -87.7321) -> (-38, -87.7321)
  line L2947 (-26, -87.7321) -> (-25.5, -86.866)
  line L2948 (-24.5, -86.866) -> (-24, -87.7321)
  line L2949 (-17, -83) -> (-18, -83)
  line L2950 (-17, -87.7321) -> (-16.5, -86.866)
  line L2951 (-17, -86) -> (-18, -86)
  line L2952 (-36, -86) -> (-36.5, -86.866)
  line L2953 (-24, -86) -> (-24.5, -86.866)
  line L2954 (-18, -87.7321) -> (-17, -87.7321)
  line L2955 (-32, -86) -> (-33, -86)
  line L2956 (-16.5, -83.866) -> (-17, -83)
  line L2957 (-18, -84.7321) -> (-17, -84.7321)
  line L2958 (-33.5, -86.866) -> (-33, -87.7321)
  line L2959 (-29, -86) -> (-30, -86)
  line L2960 (-30, -87.7321) -> (-29, -87.7321)
  line L2961 (-21, -84.7321) -> (-20, -84.7321)
  line L2962 (-32, -87.7321) -> (-31.5, -86.866)
  line L2963 (-21, -83) -> (-21.5, -83.866)
  line L2964 (-28.5, -83.866) -> (-29, -83)
  line L2965 (-29, -84.7321) -> (-28.5, -83.866)
  line L2966 (-32, -83) -> (-33, -83)
  line L2967 (-18.5, -86.866) -> (-18, -87.7321)
  line L2968 (-30, -84.7321) -> (-29, -84.7321)
  line L2969 (-30, -86) -> (-30.5, -86.866)
  line L2970 (-33, -84.7321) -> (-32, -84.7321)
  line L2971 (-11, -87.7321) -> (-10.5, -86.866)
  line L2972 (-21, -87.7321) -> (-20, -87.7321)
  line L2973 (-11, -86) -> (-12, -86)
  line L2974 (-31.5, -86.866) -> (-32, -86)
  line L2975 (-23, -84.7321) -> (-22.5, -83.866)
  line L2976 (-12, -83) -> (-12.5, -83.866)
  line L2977 (-33, -83) -> (-33.5, -83.866)
  line L2978 (-11, -84.7321) -> (-10.5, -83.866)
  line L2979 (-30.5, -83.866) -> (-30, -84.7321)
  line L2980 (-19.5, -83.866) -> (-20, -83)
  line L2981 (-33.5, -83.866) -> (-33, -84.7321)
  line L2982 (-21.5, -86.866) -> (-21, -87.7321)
  line L2983 (-18, -83) -> (-18.5, -83.866)
  line L2984 (-21, -86) -> (-21.5, -86.866)
  line L2985 (-11, -83) -> (-12, -83)
  line L2986 (-20, -87.7321) -> (-19.5, -86.866)
  line L2987 (-33, -87.7321) -> (-32, -87.7321)
  line L2988 (-20, -84.7321) -> (-19.5, -83.866)
  line L2989 (-19.5, -86.866) -> (-20, -86)
  line L2990 (-29, -83) -> (-30, -83)
  line L2991 (-30, -83) -> (-30.5, -83.866)
  line L2992 (-18, -86) -> (-18.5, -86.866)
  line L2993 (-28.5, -86.866) -> (-29, -86)
  line L2994 (-22.5, -83.866) -> (-23, -83)
  line L2995 (-20, -83) -> (-21, -83)
  line L2996 (-29, -87.7321) -> (-28.5, -86.866)
  line L2997 (-30.5, -86.866) -> (-30, -87.7321)
  line L2998 (-22.5, -86.866) -> (-23, -86)
  line L2999 (-12, -87.7321) -> (-11, -87.7321)
  line L3000 (-10.5, -86.866) -> (-11, -86)
  line L3001 (-10.5, -83.866) -> (-11, -83)
  line L3002 (-23, -87.7321) -> (-22.5, -86.866)
  line L3003 (-14, -84.7321) -> (-13.5, -83.866)
  line L3004 (-20, -86) -> (-21, -86)
  line L3005 (-12, -84.7321) -> (-11, -84.7321)
  line L3006 (-32, -84.7321) -> (-31.5, -83.866)
  line L3007 (-21.5, -83.866) -> (-21, -84.7321)
  line L3008 (-15, -87.7321) -> (-14, -87.7321)
  line L3009 (-12.5, -86.866) -> (-12, -87.7321)
  line L3010 (-12.5, -83.866) -> (-12, -84.7321)
  line L3011 (-24, -84.7321) -> (-23, -84.7321)
  line L3012 (-14, -86) -> (-15, -86)
  line L3013 (-23, -86) -> (-24, -86)
  line L3014 (-24, -87.7321) -> (-23, -87.7321)
  line L3015 (-12, -86) -> (-12.5, -86.866)
  line L3016 (-23, -83) -> (-24, -83)
  line L3017 (-14, -87.7321) -> (-13.5, -86.866)
  line L3018 (-13.5, -86.866) -> (-14, -86)
  line L3019 (-13.5, -83.866) -> (-14, -83)
  line L3020 (-14, -83) -> (-15, -83)
  line L3021 (-15, -84.7321) -> (-14, -84.7321)
  line L3022 (-60, -84.7321) -> (-59, -84.7321)
  line L3023 (-63.5, -83.866) -> (-63, -84.7321)
  line L3024 (-59, -86) -> (-60, -86)
  line L3025 (-63, -84.7321) -> (-62, -84.7321)
  line L3026 (-63, -86) -> (-63.5, -86.866)
  line L3027 (-62, -87.7321) -> (-61.5, -86.866)
  line L3028 (-62, -86) -> (-63, -86)
  line L3029 (-62, -84.7321) -> (-61.5, -83.866)
  line L3030 (-56, -84.7321) -> (-55.5, -83.866)
  line L3031 (-50, -87.7321) -> (-49.5, -86.866)
  line L3032 (-53, -87.7321) -> (-52.5, -86.866)
  line L3033 (-60.5, -83.866) -> (-60, -84.7321)
  line L3034 (-57, -83) -> (-57.5, -83.866)
  line L3035 (-55.5, -83.866) -> (-56, -83)
  line L3036 (-57, -86) -> (-57.5, -86.866)
  line L3037 (-60, -87.7321) -> (-59, -87.7321)
  line L3038 (-58.5, -83.866) -> (-59, -83)
  line L3039 (-49.5, -86.866) -> (-50, -86)
  line L3040 (-54, -86) -> (-54.5, -86.866)
  line L3041 (-66, -86) -> (-66.5, -86.866)
  line L3042 (-54, -83) -> (-54.5, -83.866)
  line L3043 (-56, -86) -> (-57, -86)
  line L3044 (-65, -86) -> (-66, -86)
  line L3045 (-54.5, -83.866) -> (-54, -84.7321)
  line L3046 (-56, -87.7321) -> (-55.5, -86.866)
  line L3047 (-62, -83) -> (-63, -83)
  line L3048 (-63, -87.7321) -> (-62, -87.7321)
  line L3049 (-61.5, -83.866) -> (-62, -83)
  line L3050 (-68, -83) -> (-69, -83)
  line L3051 (-50, -83) -> (-51, -83)
  line L3052 (-60, -86) -> (-60.5, -86.866)
  line L3053 (-58.5, -86.866) -> (-59, -86)
  line L3054 (-57.5, -86.866) -> (-57, -87.7321)
  line L3055 (-52.5, -83.866) -> (-53, -83)
  line L3056 (-69.5, -83.866) -> (-69, -84.7321)
  line L3057 (-63, -83) -> (-63.5, -83.866)
  line L3058 (-49.5, -83.866) -> (-50, -83)
  line L3059 (-65, -84.7321) -> (-64.5, -83.866)
  line L3060 (-68, -87.7321) -> (-67.5, -86.866)
  line L3061 (-57, -84.7321) -> (-56, -84.7321)
  line L3062 (-52.5, -86.866) -> (-53, -86)
  line L3063 (-51.5, -86.866) -> (-51, -87.7321)
  line L3064 (-66, -87.7321) -> (-65, -87.7321)
  line L3065 (-60.5, -86.866) -> (-60, -87.7321)
  line L3066 (-54.5, -86.866) -> (-54, -87.7321)
  line L3067 (-51, -86) -> (-51.5, -86.866)
  line L3068 (-68, -86) -> (-69, -86)
  line L3069 (-66, -84.7321) -> (-65, -84.7321)
  line L3070 (-51, -83) -> (-51.5, -83.866)
  line L3071 (-67.5, -86.866) -> (-68, -86)
  line L3072 (-54, -87.7321) -> (-53, -87.7321)
  line L3073 (-51, -84.7321) -> (-50, -84.7321)
  line L3074 (-64.5, -86.866) -> (-65, -86)
  line L3075 (-51.5, -83.866) -> (-51, -84.7321)
  line L3076 (-66.5, -83.866) -> (-66, -84.7321)
  line L3077 (-65, -83) -> (-66, -83)
  line L3078 (-64.5, -83.866) -> (-65, -83)
  line L3079 (-50, -84.7321) -> (-49.5, -83.866)
  line L3080 (-50, -86) -> (-51, -86)
  line L3081 (-65, -87.7321) -> (-64.5, -86.866)
  line L3082 (-51, -87.7321) -> (-50, -87.7321)
  line L3083 (-69, -84.7321) -> (-68, -84.7321)
  line L3084 (-53, -84.7321) -> (-52.5, -83.866)
  line L3085 (-69, -86) -> (-69.5, -86.866)
  line L3086 (-53, -86) -> (-54, -86)
  line L3087 (-67.5, -83.866) -> (-68, -83)
  line L3088 (-53, -83) -> (-54, -83)
  line L3089 (-46.5, -83.866) -> (-47, -83)
  line L3090 (-69, -87.7321) -> (-68, -87.7321)
  line L3091 (-46.5, -86.866) -> (-47, -86)
  line L3092 (-48.5, -83.866) -> (-48, -84.7321)
  line L3093 (-48, -87.7321) -> (-47, -87.7321)
  line L3094 (-45, -86) -> (-45.5, -86.866)
  line L3095 (-44, -87.7321) -> (-43.5, -86.866)
  line L3096 (-69, -83) -> (-69.5, -83.866)
  line L3097 (-48, -86) -> (-48.5, -86.866)
  line L3098 (-48, -84.7321) -> (-47, -84.7321)
  line L3099 (-45.5, -83.866) -> (-45, -84.7321)
  line L3100 (-45.5, -86.866) -> (-45, -87.7321)
  line L3101 (-66.5, -86.866) -> (-66, -87.7321)
  line L3102 (-47, -83) -> (-48, -83)
  line L3103 (-47, -87.7321) -> (-46.5, -86.866)
  line L3104 (-48.5, -86.866) -> (-48, -87.7321)
  line L3105 (-48, -83) -> (-48.5, -83.866)
  line L3106 (-54, -84.7321) -> (-53, -84.7321)
  line L3107 (-69.5, -86.866) -> (-69, -87.7321)
  line L3108 (-47, -86) -> (-48, -86)
  line L3109 (-45, -83) -> (-45.5, -83.866)
  line L3110 (-66, -83) -> (-66.5, -83.866)
  line L3111 (-47, -84.7321) -> (-46.5, -83.866)
  line L3112 (-68, -84.7321) -> (-67.5, -83.866)
  line L3113 (-40.5, -83.866) -> (-41, -83)
  line L3114 (-60, -83) -> (-60.5, -83.866)
  line L3115 (-57, -87.7321) -> (-56, -87.7321)
  line L3116 (-57.5, -83.866) -> (-57, -84.7321)
  line L3117 (-63.5, -86.866) -> (-63, -87.7321)
  line L3118 (-55.5, -86.866) -> (-56, -86)
  line L3119 (-59, -87.7321) -> (-58.5, -86.866)
  line L3120 (-56, -83) -> (-57, -83)
  line L3121 (-61.5, -86.866) -> (-62, -86)
  line L3122 (-59, -83) -> (-60, -83)
  line L3123 (-59, -84.7321) -> (-58.5, -83.866)
  line L3124 (-59, -90.7321) -> (-58.5, -89.866)
  line L3125 (-57.5, -89.866) -> (-57, -90.7321)
  line L3126 (-60, -90.7321) -> (-59, -90.7321)
  line L3127 (-54, -89) -> (-54.5, -89.866)
  line L3128 (-62, -90.7321) -> (-61.5, -89.866)
  line L3129 (-56, -90.7321) -> (-55.5, -89.866)
  line L3130 (-60.5, -89.866) -> (-60, -90.7321)
  line L3131 (-49.5, -89.866) -> (-50, -89)
  line L3132 (-51, -90.7321) -> (-50, -90.7321)
  line L3133 (-68, -90.7321) -> (-67.5, -89.866)
  line L3134 (-67.5, -89.866) -> (-68, -89)
  line L3135 (-66, -90.7321) -> (-65, -90.7321)
  line L3136 (-53, -90.7321) -> (-52.5, -89.866)
  line L3137 (-51, -89) -> (-51.5, -89.866)
  line L3138 (-65, -90.7321) -> (-64.5, -89.866)
  line L3139 (-57, -90.7321) -> (-56, -90.7321)
  line L3140 (-51.5, -89.866) -> (-51, -90.7321)
  line L3141 (-69.5, -89.866) -> (-69, -90.7321)
  line L3142 (-54.5, -89.866) -> (-54, -90.7321)
  line L3143 (-65, -89) -> (-66, -89)
  line L3144 (-69, -89) -> (-69.5, -89.866)
  line L3145 (-42, -89) -> (-42.5, -89.866)
  line L3146 (-40.5, -89.866) -> (-41, -89)
  line L3147 (-44, -89) -> (-45, -89)
  line L3148 (-16.5, -89.866) -> (-17, -89)
  line L3149 (-10.5, -89.866) -> (-11, -89)
  line L3150 (-43.5, -89.866) -> (-44, -89)
  line L3151 (-18.5, -89.866) -> (-18, -90.7321)
  line L3152 (-41, -90.7321) -> (-40.5, -89.866)
  line L3153 (-13.5, -89.866) -> (-14, -89)
  line L3154 (-12.5, -89.866) -> (-12, -90.7321)
  line L3155 (-18, -89) -> (-18.5, -89.866)
  line L3156 (-41, -89) -> (-42, -89)
  line L3157 (-12, -90.7321) -> (-11, -90.7321)
  line L3158 (-17, -89) -> (-18, -89)
  line L3159 (-14, -90.7321) -> (-13.5, -89.866)
  line L3160 (-42.5, -89.866) -> (-42, -90.7321)
  line L3161 (-17, -90.7321) -> (-16.5, -89.866)
  line L3162 (-11, -90.7321) -> (-10.5, -89.866)
  line L3163 (-15, -89) -> (-15.5, -89.866)
  line L3164 (-12, -89) -> (-12.5, -89.866)
  line L3165 (-45, -90.7321) -> (-44, -90.7321)
  line L3166 (-18, -90.7321) -> (-17, -90.7321)
  line L3167 (-11, -89) -> (-12, -89)
  line L3168 (-44, -90.7321) -> (-43.5, -89.866)
  line L3169 (-15.5, -89.866) -> (-15, -90.7321)
  line L3170 (-39.5, -89.866) -> (-39, -90.7321)
  line L3171 (-30, -90.7321) -> (-29, -90.7321)
  line L3172 (-37.5, -89.866) -> (-38, -89)
  line L3173 (-35, -89) -> (-36, -89)
  line L3174 (-32, -89) -> (-33, -89)
  line L3175 (-29, -89) -> (-30, -89)
  line L3176 (-35, -90.7321) -> (-34.5, -89.866)
  line L3177 (-31.5, -89.866) -> (-32, -89)
  line L3178 (-33, -90.7321) -> (-32, -90.7321)
  line L3179 (-29, -90.7321) -> (-28.5, -89.866)
  line L3180 (-36, -90.7321) -> (-35, -90.7321)
  line L3181 (-30.5, -89.866) -> (-30, -90.7321)
  line L3182 (-34.5, -89.866) -> (-35, -89)
  line L3183 (-38, -90.7321) -> (-37.5, -89.866)
  line L3184 (-33, -89) -> (-33.5, -89.866)
  line L3185 (-36, -89) -> (-36.5, -89.866)
  line L3186 (-39, -90.7321) -> (-38, -90.7321)
  line L3187 (-30, -89) -> (-30.5, -89.866)
  line L3188 (-38, -89) -> (-39, -89)
  line L3189 (-39, -89) -> (-39.5, -89.866)
  line L3190 (-33.5, -89.866) -> (-33, -90.7321)
  line L3191 (-45, -89) -> (-45.5, -89.866)
  line L3192 (-32, -90.7321) -> (-31.5, -89.866)
  line L3193 (-36.5, -89.866) -> (-36, -90.7321)
  line L3194 (-28.5, -89.866) -> (-29, -89)
  line L3195 (-50, -89) -> (-51, -89)
  line L3196 (-64.5, -89.866) -> (-65, -89)
  line L3197 (-66.5, -89.866) -> (-66, -90.7321)
  line L3198 (-66, -89) -> (-66.5, -89.866)
  line L3199 (-46.5, -89.866) -> (-47, -89)
  line L3200 (-52.5, -89.866) -> (-53, -89)
  line L3201 (-50, -90.7321) -> (-49.5, -89.866)
  line L3202 (-69, -90.7321) -> (-68, -90.7321)
  line L3203 (-54, -90.7321) -> (-53, -90.7321)
  line L3204 (-68, -89) -> (-69, -89)
  line L3205 (-53, -89) -> (-54, -89)
  line L3206 (-57, -89) -> (-57.5, -89.866)
  line L3207 (-63.5, -89.866) -> (-63, -90.7321)
  line L3208 (-55.5, -89.866) -> (-56, -89)
  line L3209 (-61.5, -89.866) -> (-62, -89)
  line L3210 (-59, -89) -> (-60, -89)
  line L3211 (-56, -89) -> (-57, -89)
  line L3212 (-62, -89) -> (-63, -89)
  line L3213 (-63, -89) -> (-63.5, -89.866)
  line L3214 (-58.5, -89.866) -> (-59, -89)
  line L3215 (-63, -90.7321) -> (-62, -90.7321)
  line L3216 (-60, -89) -> (-60.5, -89.866)
  line L3217 (-21.5, -89.866) -> (-21, -90.7321)
  line L3218 (-20, -89) -> (-21, -89)